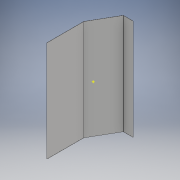
# Autodesk Inventor part: Front Cover with Cent point
Saved by Autodesk Inventor 2018 (Build 220112000, 112)
## iProperties
Created: 2018-06-12
Part Number: Front Cover with Cent point
Material: Copper
Document SubType Name: Sheet Metal
Designer: p446024
Mass: 17309.3 g
Surface Area: 24272.8 cm^2
Volume: 1936.17 cm^3
Density: 8.94 g/cm^3
Sheet Metal Rule: Default_mm
Appearance: Default
Author: p446024
Autodesk Inventor part; units mm, degrees
ref_plane "YZ Plane" through (0, 0, 0) normal (1, 0, 0) x (0, 1, 0)
ref_plane "XZ Plane" through (0, 0, 0) normal (0, 1, 0) x (-1, 0, 0)
ref_plane "XY Plane" through (0, 0, 0) normal (0, 0, 1) x (1, 0, 0)
sketch "Sketch1" plane through (0, 0, 0) normal (0, 0, 1) x (1, 0, 0)
  line L0 (0, 0) -> (0, 440)
  line L1 (0, 440) -> (172.5, 738.7788)
  line L2 (172.5, 738.7788) -> (289.5, 738.7788)
  dimension "d0" = 440
  dimension "d1" = 345
  dimension "d2" = 150
  dimension "d3" = 117
  measures "d0" distance of L0.start L0.end
  measures "d1" distance of L0.end L1.end
  measures "d2" angle of L0 L1
  measures "d3" distance of L1.end L2.end
contour flange "Contour Flange1" sketch "Sketch1" thickness 1.6 bend radius 1.6 width 1200 along (0, 0, 1) mid plane no both sides no wall seen from (0, 220, 0) lies toward (1, 0, 0) curves L0 L1 L2
bend "Bend1"
corner "Corner1"
equation "\"d4\" = Thickness"
equation "\"d5\" = BendReliefWidth"
equation "\"d6\" = BendReliefDepth"
equation "\"d7\" = MinimumRemnant"
equation "\"d8\" = TransitionRadius"
equation "\"d10\" = BendRadius"
equation "\"d12\" = CornerReliefSize"
equation "\"d13\" = GapSize"
equation "\"d14\" = JacobiRadiusSize"
equation "\"BendRadius\" = Thickness"
equation "\"BendReliefWidth\" = Thickness"
equation "\"BendReliefDepth\" = 0.5 * Thickness"
equation "\"CornerReliefSize\" = 4 * Thickness"
equation "\"MinimumRemnant\" = 2 * Thickness"
equation "\"TransitionRadius\" = BendRadius"
equation "\"JacobiRadiusSize\" = BendRadius"
equation "\"GapSize\" = Thickness"
equation "\"Thickness\" = 1.6"
body "Solid1"
